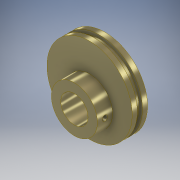
# Autodesk Inventor part: reverse gear eccentric 1
Saved by Autodesk Inventor 2017 (Build 210142000, 142)
## iProperties
Created: 2018-11-07
Part Number: reverse gear eccentric 1
Material: Generic
Document SubType Name: Modeling
Designer: User
Density: 1 g/cm^3
Appearance: Default
Author: User
Autodesk Inventor part; units mm, degrees
ref_plane "XZ Plane" through (0, 0, 0) normal (0, 1, 0) x (-1, 0, 0)
ref_plane "XY Plane" through (0, 0, 0) normal (0, 0, 1) x (1, 0, 0)
sketch "Sketch1" plane through (0, 0, 0) normal (0, 1, 0) x (-1, 0, 0)
  circle A0 centre (0, 0) radius 11.5
  dimension "d0" = 23
  constraints: 1 centre point, 1 coincident
  measures "d0" diameter of A0
extrude "Extrusion1" add sketch "Sketch1" along normal blind 1.5
sketch "Sketch2" plane through (0, 1.5, 0) normal (0, 1, 0) x (1, 0, 0)
  circle A0 centre (0, 0) radius 12.5
  dimension "d3" = 25
  constraints: 1 centre point, 1 coincident
  measures "d3" diameter of A0
extrude "Extrusion2" add sketch "Sketch2" along normal blind 1.5
sketch "Sketch3" plane through (0, 0, 0) normal (0, -1, 0) x (1, 0, 0)
  circle A0 centre (0, 0) radius 12.5
  dimension "d6" = 25
  constraints: 1 centre point, 1 coincident
  measures "d6" diameter of A0
extrude "Extrusion3" add sketch "Sketch3" along normal blind 1.5
sketch "Sketch4" plane through (0, -1.5, 0) normal (0, -1, 0) x (1, 0, 0)
  circle A0 centre (0, 0) radius 12.5 projected
  line L0 (0, -12.5) -> (0, -9.5) construction
  circle A1 centre (0, -2.6096) radius 6.75
  circle A2 centre (0, -2.6096) radius 4
  dimension "d9" = 3
  dimension "d17" = 13.5
  dimension "d18" = 8
  constraints: 2 centre point, 2 end point, 1 coincident, 1 vertical, 1 vertical alignment, 1 other
  measures "d9" distance of L0.start L0.end
  measures "d17" diameter of A1
  measures "d18" diameter of A2
extrude "Extrusion6" add sketch "Sketch4" along normal blind 4.45 contours A1
extrude "Extrusion7" cut sketch "Sketch4" against normal blind 10 contours A2
ref_plane "Work Plane1" through (6.76, 0, 0) normal (1, 0, 0) x (0, 1, 0)
sketch "Sketch6" plane through (6.76, 0, 0) normal (1, 0, 0) x (0, 1, 0)
  line L0 (-5.95, 4.1404) -> (-5.95, -9.3596) projected
  line L1 (-1.5, -9.3596) -> (-1.5, 4.1404) projected
  line L2 (-5.95, -9.3596) -> (-5.95, 4.1404) construction
  line L3 (-1.5, -9.3596) -> (-5.95, -9.3596) construction
  line L4 (-5.95, 4.1404) -> (-1.5, 4.1404) construction
  line L5 (-1.5, 4.1404) -> (-5.95, 4.1404) construction
  line L6 (-5.95, -9.3596) -> (-5.95, -2.6096) construction
  line L7 (-5.95, 4.1404) -> (-3.725, 4.1404) construction
  line L8 (-3.725, 3.1248) -> (-3.725, -6.8752) construction
  circle A0 centre (-3.725, -2.6096) radius 0.8
  point P0 (0, 0)
  dimension "d24" = 4.45
  dimension "d25" = 13.5
  dimension "d26" = 6.75
  dimension "d27" = 2.225
  dimension "d28" = 10
  dimension "d29" = 1.6
  constraints: 10 end point, 2 midpoint, 1 centre point, 1 collinear, 1 perpendicular, 1 point on line, 1 vertical
  measures "d24" distance of L0.start L1.end
  measures "d25" distance of L0.start L0.end
  measures "d26" distance of L3.end L6.end
  measures "d27" distance of L5.end L7.end
  measures "d28" distance of L8.start L8.end
  measures "d29" diameter of A0
extrude "Extrusion8" cut sketch "Sketch6" against normal blind 4.45
sketch "Sketch7" plane through (0, 3, 0) normal (0, 1, 0) x (1, 0, 0)
  circle A0 centre (0, 0) radius 11
  circle A1 centre (0, 2.6096) radius 4 projected
  circle A2 centre (0, 2.6096) radius 4
  dimension "d32" = 22
  constraints: 2 centre point, 2 coincident
  measures "d32" diameter of A0
extrude "Extrusion10" add sketch "Sketch7" along normal blind 0.2
body "Solid1"
